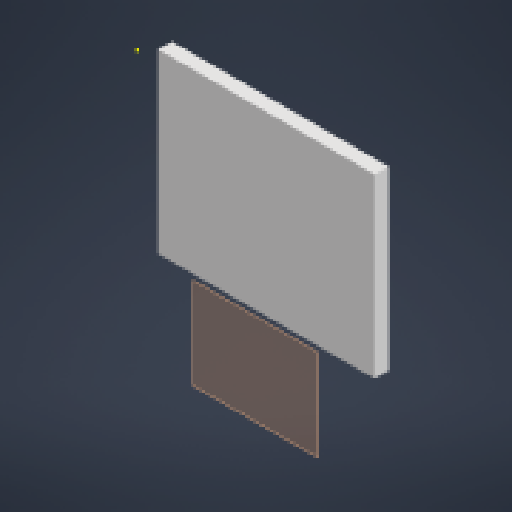
# Autodesk Inventor part: batteryFlap
Saved by Autodesk Inventor 2027 (Build 310192000, 192)
## iProperties
Created: 2026-04-18
Part Number: batteryFlap
Material: Generic
Document SubType Name: Modeling
Designer: bwalt
Density: 1 g/cm^3
Appearance: Default
Author: bwalt
Autodesk Inventor part; units mm, degrees
ref_plane "YZ Plane" through (0, 0, 0) normal (1, 0, 0) x (0, 1, 0)
ref_plane "XZ Plane" through (0, 0, 0) normal (0, 1, 0) x (-1, 0, 0)
ref_plane "XY Plane" through (0, 0, 0) normal (0, 0, 1) x (1, 0, 0)
ref_plane "Work Plane6" through (39.7008, -57.1298, -11.5364) normal (0, 0, 1) x (1, 0, 0)
sketch "Sketch1" plane through (39.7008, -57.1298, -11.5364) normal (0, 0, 1) x (1, 0, 0)
  line L0 (-30.146, 63.9369) -> (29.7552, 63.9369)
  line L1 (29.7552, 63.9369) -> (29.7552, 15.006)
  line L2 (29.7552, 15.006) -> (-30.146, 15.006)
  line L3 (-30.146, 15.006) -> (-30.146, 63.9369)
  point P0 (-39.7008, 57.1298)
  constraints: 8 end point, 2 parallel, 1 horizontal, 1 perpendicular
extrude "Extrusion1" add sketch "Sketch1" against normal blind 3.81
ref_plane "Work Plane5" through (9.5547, -42.1238, -11.5364) normal (0, -1, 0) x (1, 0, 0)
sketch "Sketch4" plane through (9.5547, -42.1238, -11.5364) normal (0, -1, 0) x (1, 0, 0)
  line L0 (59.9013, -3.81) -> (0, -3.81) projected
  line L1 (51.9539, -3.81) -> (48.6512, -3.81)
  line L2 (48.6512, -3.81) -> (48.6512, -2.9224)
  line L3 (48.6512, -2.9224) -> (51.9539, -2.9224)
  line L4 (51.9539, -2.9224) -> (51.9539, -3.81)
  line L5 (14.0976, -3.7678) -> (10.0617, -3.7678)
  line L6 (10.0617, -3.7678) -> (10.0617, -2.9224)
  line L7 (10.0617, -2.9224) -> (14.0976, -2.9224)
  line L8 (14.0976, -2.9224) -> (14.0976, -3.7678)
  point P0 (-9.5547, 11.5364)
  point P1 (48.6512, -3.81)
  constraints: 16 end point, 4 parallel, 2 horizontal, 2 perpendicular, 2 point on line
extrude "Extrusion2" add sketch "Sketch4" along normal blind 2.54
sketch "Sketch5" plane through (39.7008, -57.1298, -11.5364) normal (0, 0, 1) x (1, 0, 0)
  line L0 (-17.172, 70.4399) -> (-9.7142, 70.4399)
  line L1 (-9.7142, 70.4399) -> (-9.7142, 57.1298)
  line L2 (-9.7142, 57.1298) -> (-17.172, 57.1298)
  line L3 (-17.172, 57.1298) -> (-17.172, 70.4399)
  point P0 (-39.7008, 57.1298)
  constraints: 8 end point, 2 parallel, 1 horizontal, 1 perpendicular
extrude "Extrusion3" add sketch "Sketch5" along normal blind 2.54
body "Solid1"
